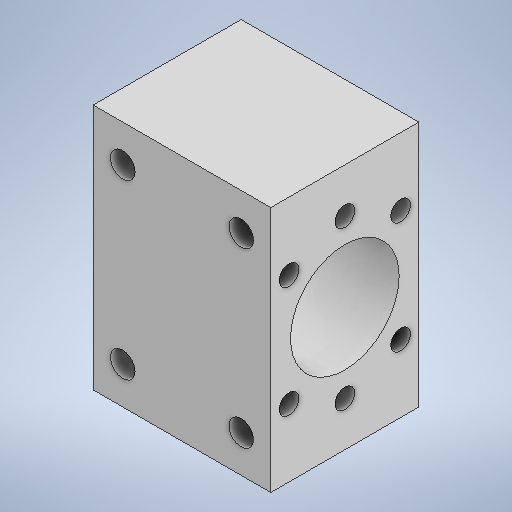
# Autodesk Inventor part: DSG12H - TO_MS_SPEC
Saved by Autodesk Inventor 2025.2 (Build 292293000, 293)
## iProperties
Created: 2026-02-05
Part Number: DSG12H - TO_MS_SPEC
Material: Generic
Document SubType Name: Modeling
Designer: composite
Density: 1 g/cm^3
Appearance: Default
Author: composite
Autodesk Inventor part; units mm, degrees
ref_plane "YZ Plane" through (0, 0, 0) normal (1, 0, 0) x (0, 1, 0)
ref_plane "XZ Plane" through (0, 0, 0) normal (0, 1, 0) x (-1, 0, 0)
ref_plane "XY Plane" through (0, 0, 0) normal (0, 0, 1) x (1, 0, 0)
sketch "Sketch1" plane through (0, 0, 0) normal (1, 0, 0) x (0, 1, 0)
  line L0 (0, 0) -> (50, 0)
  line L1 (50, 0) -> (50, -30)
  line L2 (50, -30) -> (0, -30)
  line L3 (0, -30) -> (0, 0)
  line L4 (50, 0) -> (0, -30) construction
  line L5 (0, 0) -> (50, -30) construction
  circle A0 centre (25, -15) radius 11
  dimension "d0" = 30
  dimension "d1" = 50
  dimension "d2" = 22
  constraints: 12 end point, 2 parallel, 1 centre point, 1 horizontal, 1 midpoint, 1 perpendicular
  measures "d0" distance of L0.end L1.end
  measures "d1" distance of L1.end L2.end
  measures "d2" diameter of A0
extrude "Extrusion1" add sketch "Sketch1" along normal blind 36
sketch "Sketch2" plane through (36, 0, 0) normal (1, 0, 0) x (0, 0, -1)
  circle A0 centre (15, 25) radius 11 projected
  circle A1 centre (15, 25) radius 16 construction
  circle A2 centre (15, 41) radius 2
  circle A3 centre (3.6863, 36.3137) radius 2
  circle A4 centre (-1, 25) radius 2
  circle A5 centre (3.6863, 13.6863) radius 2
  circle A6 centre (15, 9) radius 2
  circle A7 centre (26.3137, 13.6863) radius 2
  circle A8 centre (31, 25) radius 2
  circle A9 centre (26.3137, 36.3137) radius 2
  point P0 (0, 0)
  dimension "d5" = 32
  dimension "d6" = 4
  dimension "d9" = 360
  constraints: 8 centre point, 2 vertical alignment, 1 coincident, 19 other
  measures "d6" diameter of A2
extrude "Extrusion2" cut sketch "Sketch2" against normal blind 10 contours A2 | A3 | A5 | A6 | A7 | A9
sketch "Sketch3" plane through (0, 0, 0) normal (0, 0, 1) x (1, 0, 0)
  circle A0 centre (6, 42.5) radius 2.5
  circle A1 centre (30, 42.5) radius 2.5
  circle A2 centre (6, 7.5) radius 2.5
  circle A3 centre (30, 7.5) radius 2.5
  line L0 (30, 42.5) -> (30, 7.5) construction
  line L1 (36, 50) -> (36, 0) projected
  point P0 (0, 0)
  point P1 (30, 25)
  point P2 (36, 25)
  dimension "d13" = 5
  dimension "d14" = 6
  dimension "d16" = 24
  dimension "d17" = 35
  constraints: 4 centre point, 3 equal radius, 3 horizontal alignment, 2 end point, 2 midpoint, 2 vertical alignment, 1 vertical
  measures "d13" diameter of A0
  measures "d14" horizontal distance of A2.centre point (0, 0)
  measures "d16" distance of L0.end A2.centre
  measures "d17" distance of L0.start L0.end
extrude "Extrusion3" cut sketch "Sketch3" against normal blind 10
body "Solid1"
